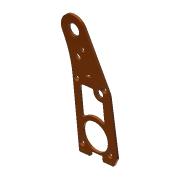
# Autodesk Inventor part: UPPER_LEG_MIDDLE_FRAME_2
Saved by Autodesk Inventor 2019.4 (Build 234330000, 330)
## iProperties
Created: 2019-11-14
Part Number: UPPER_LEG_MIDDLE_FRAME_2
Material: 一般
Document SubType Name: Modeling
Designer: y6tada
Density: 1 g/cm^3
Appearance: 滑らか - 淡いオレンジ
Author: y6tada
Autodesk Inventor part; units mm, degrees
ref_plane "YZ Plane" through (0, 0, 0) normal (1, 0, 0) x (0, 1, 0)
ref_plane "XZ Plane" through (0, 0, 0) normal (0, 1, 0) x (-1, 0, 0)
ref_plane "XY Plane" through (0, 0, 0) normal (0, 0, 1) x (1, 0, 0)
sketch "スケッチ1" plane through (0, 0, 0) normal (0, 0, 1) x (1, 0, 0)
  line L0 (0, 0) -> (-7.8332, 74.5283) construction
  line L1 (0, 0) -> (0, 134.5604) construction
  circle A0 centre (-16.8762, 26.6318) radius 1 construction
  circle A1 centre (10.9704, 29.5586) radius 1 construction
  line L2 (3.0524, 29.3154) -> (3.3227, 26.7438) projected
  arc A2 (3.0524, 29.3154) -> (1.4981, 30.5741) centre (2.2753, 29.9448) ccw projected
  arc A3 (-7.8221, 29.5945) -> (-9.0807, 28.0402) centre (-8.4514, 28.8173) ccw projected
  line L3 (-8.8105, 25.4686) -> (-9.0807, 28.0402) projected
  line L4 (13.9144, 27.8571) -> (7.5904, 88.0256) construction
  line L5 (13.9144, 27.8571) -> (28.9995, 61.7387)
  line L6 (-8.8105, 25.4686) -> (-9.2555, 24.9191)
  line L7 (-9.2555, 24.9191) -> (-18.8526, 23.9104)
  line L8 (3.3227, 26.7438) -> (3.8722, 26.2988)
  line L9 (3.8722, 26.2988) -> (13.4694, 27.3075)
  line L10 (-7.8221, 29.5945) -> (1.4981, 30.5741)
  line L11 (3.8722, 26.2988) -> (-9.2555, 24.9191) construction
  arc A4 (-10.8792, -1.6259) -> (-18.8786, 22.5819) centre (-85.0554, -12.7116) ccw construction
  line L12 (13.9144, 27.8571) -> (13.4694, 27.3075)
  line L13 (-19.4021, 24.3553) -> (-18.8526, 23.9104)
  circle A5 centre (3.8901, 77.2154) radius 7.16 construction
  circle A6 centre (-25, 122.4745) radius 9.55 construction
  circle A7 centre (-21.2321, 104.0155) radius 2 construction
  line L14 (-15.9609, 44.2312) -> (-19.3155, 76.1481) construction
  arc A8 (-14.8655, 81.6434) -> (-19.3155, 76.1481) centre (-14.3428, 76.6708) ccw projected
  line L15 (-14.8655, 81.6434) -> (-2.434, 82.95) construction
  line L16 (3.0613, 78.5) -> (5.9572, 50.9476) construction
  line L17 (4.5173, 71.2482) -> (2.8365, 71.0716)
  line L18 (-2.077, 76.5882) -> (-2.6377, 81.9231)
  arc A9 (-2.077, 76.5882) -> (4.5173, 71.2482) centre (3.8901, 77.2154) ccw
  line L19 (-14.8655, 81.6434) -> (-3.7368, 82.8131)
  line L20 (3.9356, 70.1816) -> (4.9303, 60.7174)
  arc A10 (-2.6377, 81.9231) -> (-3.7368, 82.8131) centre (-3.6323, 81.8185) ccw
  arc A11 (3.9356, 70.1816) -> (2.8365, 71.0716) centre (2.9411, 70.077) ccw
  line L21 (-19.3155, 76.1481) -> (-17.3476, 57.4248)
  circle A12 centre (-3.7775, 43.594) radius 12 construction
  circle A13 centre (-3.7775, 43.594) radius 12.2
  arc A14 (2.2029, 58.6497) -> (-14.0859, 56.0911) centre (-3.7775, 43.594) ccw
  arc A15 (2.2029, 58.6497) -> (4.9303, 60.7174) centre (2.9413, 60.5084) ccw
  arc A16 (-17.3476, 57.4248) -> (-14.0859, 56.0911) centre (-15.3585, 57.6339) ccw
  circle A17 centre (-22.3632, 83.6205) radius 1.3 construction
  circle A18 centre (4.4889, 86.4428) radius 1.3 construction
  circle A19 centre (9.9243, 34.7276) radius 1.3 construction
  circle A20 centre (-16.9277, 31.9053) radius 1.3 construction
  circle A21 centre (-15.447, 110.9099) radius 2.05 projected
  arc A22 (-21.785, 101.8583) -> (-19.4333, 105.2168) centre (-20.6092, 103.5375) ccw projected
  arc A23 (-19.6004, 105.3375) -> (-19.4333, 105.2168) centre (-15.447, 110.9099) ccw construction
  arc A24 (-20.3614, 105.9955) -> (-23.2605, 103.0964) centre (-21.8109, 104.5459) ccw projected
  arc A25 (-23.2605, 103.0964) -> (-21.785, 101.8583) centre (-15.447, 110.9099) ccw projected
  arc A26 (-20.3614, 105.9955) -> (-19.4333, 105.2168) centre (-15.447, 110.9099) ccw
  arc A27 (-15.447, 91.9599) -> (-12.1564, 92.2478) centre (-15.447, 110.9099) ccw projected
  arc A28 (-11.7917, 90.1797) -> (-12.1564, 92.2478) centre (-11.974, 91.2137) ccw projected
  arc A29 (-15.447, 89.8599) -> (-11.7917, 90.1797) centre (-15.447, 110.9099) ccw projected
  arc A30 (-15.447, 91.9599) -> (-15.447, 89.8599) centre (-15.447, 90.9099) ccw projected
  line L22 (-25, 122.4745) -> (0, 0) construction
  line L23 (28.9995, 61.7387) -> (-17.9684, 153.3176)
  line L24 (-17.9684, 153.3176) -> (-45.126, 132.0122)
  line L25 (-45.126, 132.0122) -> (-19.4021, 24.3553)
  point P0 (3.8311, 71.1761)
  point P1 (-2.7423, 82.9176)
  point P2 (5.3213, 56.9974)
  point P3 (-16.8933, 53.1027)
  point P4 (-16.8933, 53.1027)
  dimension "d0" = 6
  dimension "d1" = 45
  dimension "d2" = 45
  dimension "d3" = 0.5
  dimension "d4" = 45
  dimension "d5" = 45
  dimension "d6" = 6
  dimension "d7" = 1
  dimension "d8" = 0.2
  dimension "d10" = 4
  dimension "d11" = 2
  dimension "d42" = 30
  constraints: 40 end point, 17 point on circle, 10 coincident, 10 point on line, 10 tangent, 8 centre point, 4 collinear, 4 perpendicular, 2 equal radius, 1 concentric, 1 vertical
  measures "d0" angle of L0 L1
  measures "d1" angle of L8 L2
  measures "d2" angle of L6 L3
  measures "d3" distance from line of L9 L2.end
  measures "d4" angle of L7 L13
  measures "d5" angle of L9 L12
  measures "d6" radius of A9
  measures "d7" radius of A10
  measures "d8" radial gap between concentric circles of A12 A13
  measures "d10" radial gap between concentric circles of A14 A13
  measures "d11" radius of A15
  measures "d42" angle of L4 L5
extrude "押し出し1" add sketch "スケッチ1" against normal blind 2
hole "穴1" at (10.9704, 29.5586, 0) at (-16.8762, 26.6318, 0) direction (0, 0, -1) diameter 2 end through all
hole "穴2" at (9.9243, 34.7276, 0) at (4.4889, 86.4428, 0) at (-22.3632, 83.6205, 0) at (-16.9277, 31.9053, 0) direction (0, 0, -1) diameter 2.6 end through all countersink diameter 5.5 countersink angle 90 clearance for "Countersunk Flat Head Screw ISO 2009/7046" size "M2.5" standard "ISO"
hole "穴3" at (-25, 122.4745, 0) direction (0, 0, -1) diameter 10 end through all counterbore diameter 11.3 counterbore depth 0.65
hole "穴4" at (3.8901, 77.2154, 0) direction (0, 0, -1) diameter 6 end through all counterbore diameter 7.3 counterbore depth 0.65
